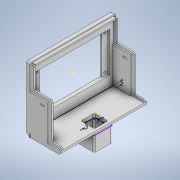
# Autodesk Inventor part: sUPORTE
Saved by Autodesk Inventor 2022 (Build 260153000, 153)
## iProperties
Created: 2022-12-13
Part Number: sUPORTE
Material: Genérico
Document SubType Name: Modeling
Designer: gugarauj07
Density: 1 g/cm^3
Appearance: Padrão
Author: gugarauj07
Autodesk Inventor part; units mm, degrees
ref_plane "YZ Plane" through (0, 0, 0) normal (1, 0, 0) x (0, 1, 0)
ref_plane "XZ Plane" through (0, 0, 0) normal (0, 1, 0) x (-1, 0, 0)
ref_plane "XY Plane" through (0, 0, 0) normal (0, 0, 1) x (1, 0, 0)
sketch "Esboço1" plane through (0, 0, 0) normal (1, 0, 0) x (0, 1, 0)
  line L0 (40.5, 60) -> (-42.5, 60)
  line L1 (-42.5, 60) -> (-42.5, -60)
  line L2 (-42.5, -60) -> (40.5, -60)
  line L3 (42.5, -58) -> (42.5, 58)
  line L4 (-42.5, 60) -> (42.5, -60) construction
  arc A0 (42.5, 58) -> (40.5, 60) centre (40.5, 58) ccw
  arc A1 (40.5, -60) -> (42.5, -58) centre (40.5, -58) ccw
  point P0 (0, 0)
  dimension "d0" = 85
  dimension "d1" = 120
  dimension "d4" = 2
  constraints: 10 end point, 4 point on circle, 4 tangent, 2 centre point, 2 parallel, 2 point on line, 1 equal radius, 1 horizontal, 1 midpoint, 1 perpendicular
  measures "d0" distance of L4.end L1.end
  measures "d1" distance of L0.end L1.end
  measures "d4" radius of A0
extrude "Extrusão1" add sketch "Esboço1" along normal blind 5
sketch "Esboço4" plane through (5, 0, 0) normal (1, 0, 0) x (0, 0, -1)
  line L0 (-60, -42.5) -> (60, -42.5) projected
  line L1 (-60, -42.5) -> (60, -42.5)
  line L2 (60, -42.5) -> (60, -47.5)
  line L3 (60, -47.5) -> (-60, -47.5)
  line L4 (-60, -47.5) -> (-60, -42.5)
  point P0 (0, 0)
  point P1 (60, -42.5)
  dimension "d33" = 5
  constraints: 8 end point, 2 parallel, 1 horizontal, 1 perpendicular
  measures "d33" distance of L1.end L2.end
extrude "Extrusão3" add sketch "Esboço4" against normal blind 5
sketch "Esboço5" plane through (5, 0, 0) normal (1, 0, 0) x (0, 0, -1)
  line L0 (-60, 40.5) -> (-60, -47.5) projected
  line L1 (60, 40.5) -> (60, -47.5) projected
  line L2 (-60, -47.5) -> (60, -47.5)
  line L3 (60, -47.5) -> (60, -42.5)
  line L4 (60, -42.5) -> (-60, -42.5)
  line L5 (-60, -42.5) -> (-60, -47.5)
  point P0 (0, 0)
  point P1 (60, -47.5)
  dimension "d36" = 5
  constraints: 8 end point, 2 parallel, 1 horizontal, 1 perpendicular, 1 point on line
  measures "d36" distance of L3.end L2.end
extrude "Extrusão4" add sketch "Esboço5" along normal blind 43
chamfer "Chanfro2" distance 4 angle 45 1 edges at (0, -47.5, 0)
chamfer "Chanfro3" distance 2 angle 45 1 edges at (48, -47.5, 0)
sketch "Esboço9" plane through (4, -47.5, -60) normal (0, -1, 0) x (1, 0, 0)
  line L0 (23.5, 50.5) -> (38.5, 50.5) projected
  line L1 (31, 50.5) -> (31, 47.5)
  line L2 (38.5, 69.5) -> (23.5, 69.5) projected
  line L3 (31, 69.5) -> (31, 72.5)
  line L4 (43.5, 72.5) -> (16.5, 72.5)
  line L5 (43.5, 47.5) -> (16.5, 47.5)
  line L6 (16.5, 47.5) -> (16.5, 72.5)
  line L7 (43.5, 72.5) -> (43.5, 47.5)
  line L8 (31, 69.5) -> (29.1751, 69.5)
  arc A0 (23.5, 69.5) -> (21.5, 67.5) centre (23.5, 67.5) ccw projected
  line L9 (31, 69.5) -> (23.5, 69.5)
  line L10 (21.5, 67.5) -> (21.5, 52.5) projected
  line L11 (21.5, 67.5) -> (21.5, 52.5)
  arc A1 (21.5, 52.5) -> (23.5, 50.5) centre (23.5, 52.5) ccw projected
  line L12 (23.5, 50.5) -> (31, 50.5)
  line L13 (31, 50.5) -> (38.5, 50.5)
  arc A2 (38.5, 50.5) -> (40.5, 52.5) centre (38.5, 52.5) ccw projected
  line L14 (40.5, 52.5) -> (40.5, 67.5)
  line L15 (38.5, 69.5) -> (31, 69.5)
  arc A3 (38.5, 50.5) -> (40.5, 52.5) centre (38.5, 52.5) ccw
  arc A4 (21.5, 52.5) -> (23.5, 50.5) centre (23.5, 52.5) ccw
  arc A5 (23.5, 69.5) -> (21.5, 67.5) centre (23.5, 67.5) ccw
  arc A6 (40.5, 67.5) -> (38.5, 69.5) centre (38.5, 67.5) ccw projected
  arc A7 (40.5, 67.5) -> (38.5, 69.5) centre (38.5, 67.5) ccw
  point P0 (-4, 60)
  dimension "d103" = 3
  dimension "d104" = 3
  constraints: 26 end point, 8 point on circle, 5 vertical, 4 centre point, 4 tangent, 3 collinear, 2 midpoint, 2 perpendicular, 1 horizontal, 1 point on line
  measures "d103" distance of L1.start L1.end
  measures "d104" distance of L3.start L3.end
extrude "Extrusão7" add sketch "Esboço9" along normal blind 21 contours L0 L1 L5 L6 L4 L3 L2 A0 L10 A1
extrude "Extrusão9" add sketch "Esboço9" along normal blind 21 contours L0 A2 L14 A6 L2 L3 L4 L7 L5 L1
fillet "Arredondamento1" radius 2 4 edges at (47.5, -58, -12.5) (20.5, -58, -12.5) (20.5, -58, 12.5) (47.5, -58, 12.5)
sketch "Esboço12" plane through (5, 0, 0) normal (1, 0, 0) x (0, 0, -1)
  line L0 (60, -42.5) -> (60, 40.5) projected
  line L1 (60, -42.5) -> (55, -42.5)
  line L2 (55, -42.5) -> (55, 7.5)
  line L3 (55, 7.5) -> (60, 7.5)
  line L4 (60, 7.5) -> (60, -42.5)
  line L5 (60, -42.5) -> (-60, -42.5) projected
  line L6 (-60, -42.5) -> (-55, -42.5)
  line L7 (-55, -42.5) -> (-55, 7.5)
  line L8 (-55, 7.5) -> (-60, 7.5)
  line L9 (-60, 7.5) -> (-60, -42.5)
  point P0 (0, 0)
  dimension "d123" = 5
  dimension "d124" = 50
  dimension "d125" = 5
  dimension "d126" = 50
  constraints: 16 end point, 4 parallel, 2 horizontal, 2 perpendicular
  measures "d123" distance of L2.end L3.end
  measures "d124" distance of L1.end L2.end
  measures "d125" distance of L8.end L7.end
  measures "d126" distance of L7.end L6.end
extrude "Extrusão10" add sketch "Esboço12" along normal blind 25
sketch "Esboço13" plane through (30, 0, 0) normal (1, 0, 0) x (0, 0, -1)
  line L0 (-60, 40.5) -> (-60, -43.5) projected
  line L1 (-60, -42.5141) -> (-58.5, -42.5141)
  line L2 (-60, -42.5141) -> (-58.5, -42.5141) construction
  line L3 (60, -42.5) -> (-60, -42.5) projected
  line L4 (-55, 7.5) -> (-60, 7.5) projected
  line L5 (-58.5, -42.5) -> (-56.5, -42.5)
  line L6 (-56.5, -42.5) -> (-56.5, 7.5)
  line L7 (-56.5, 7.5) -> (-58.5, 7.5)
  line L8 (-58.5, 7.5) -> (-58.5, -42.5)
  line L9 (58, 42.5) -> (-58, 42.5) projected
  line L10 (-57.5, 42.5) -> (-56, 42.5) construction
  line L11 (-58.5, 7.5) -> (-56.5, 7.5)
  line L12 (60, -42.5) -> (55, -42.5) projected
  line L13 (60, -42.5) -> (58.5, -42.5)
  line L14 (55, 7.5) -> (60, 7.5) projected
  line L15 (58.5, -42.5) -> (56.5, -42.5)
  line L16 (56.5, -42.5) -> (56.5, 7.5)
  line L17 (56.5, 7.5) -> (58.5, 7.5)
  line L18 (58.5, 7.5) -> (58.5, -42.5)
  point P0 (0, 0)
  dimension "d129" = 1.5
  dimension "d130" = 0
  dimension "d135" = 1.5
  dimension "d136" = 2
  constraints: 26 end point, 6 point on line, 5 horizontal, 4 parallel, 3 perpendicular, 1 collinear
  measures "d129" distance of L1.start L1.end
  measures "d130" distance between parallel lines of L1 L2
  measures "d135" distance of L3.start L13.end
  measures "d136" distance of L16.end L17.end
extrude "Extrusão11" add sketch "Esboço13" along normal blind 4 contours L4 L6 L3 L8 | L3 L16 L14 L18
extrude "Extrusão12" cut sketch "Esboço9" against normal blind 6 contours A1 L10 A0 L2 A6 L14 A2 L0
sketch "Esboço14" plane through (5, 0, 0) normal (1, 0, 0) x (0, 0, -1)
  line L0 (-58.5, 7.5) -> (-60, 7.5) projected
  line L1 (-58.5, 7.5) -> (-56.5, 7.5)
  line L2 (-56.5, 7.5) -> (-56.5, 41)
  line L3 (-56.5, 41) -> (-56.5, 41)
  line L4 (-58.5, 39) -> (-58.5, 7.5)
  line L5 (55, 7.5) -> (60, 7.5) projected
  line L6 (58.5055, 7.5) -> (56.5055, 7.5)
  line L7 (56.5055, 7.5) -> (56.5055, 41)
  line L8 (56.5055, 41) -> (56.5055, 41)
  line L9 (58.5055, 39) -> (58.5055, 7.5)
  line L10 (-56.5, 41) -> (56.5055, 41)
  line L11 (56.5055, 41) -> (56.5055, 39)
  line L12 (56.5055, 39) -> (-56.5, 39)
  line L13 (-56.5, 39) -> (-56.5, 41)
  arc A0 (-56.5, 41) -> (-58.5, 39) centre (-56.5, 39) ccw
  arc A1 (58.5055, 39) -> (56.5055, 41) centre (56.5055, 39) ccw
  point P0 (0, 0)
  point P1 (-58.5, 41)
  point P2 (58.5055, 41)
  dimension "d141" = 2
  dimension "d142" = 33.5
  dimension "d143" = 2
  dimension "d144" = 33.5
  dimension "d145" = 2
  dimension "d146" = 2
  dimension "d147" = 2
  constraints: 24 end point, 6 parallel, 6 point on line, 4 point on circle, 4 tangent, 3 horizontal, 3 perpendicular, 2 centre point
  measures "d141" distance of point (-58.5, 41) L2.end
  measures "d142" distance of L2.end L1.end
  measures "d143" distance of L7.end point (58.505, 41)
  measures "d144" distance of L6.end L7.end
  measures "d145" distance of L10.end L11.end
  measures "d146" radius of A0
  measures "d147" radius of A1
extrude "Extrusão13" add sketch "Esboço14" along normal blind 4
sketch "Esboço15" plane through (9, 0, 0) normal (1, 0, 0) x (0, 0, -1)
  line L0 (-56.5, 7.5) -> (-56.5, 39) projected
  line L1 (-56.5, 7.5) -> (-58.5, 7.5)
  line L2 (-58.5, 7.5) -> (-58.5, 10.5)
  line L3 (-58.5, 10.5) -> (-56.5, 10.5)
  line L4 (-56.5, 10.5) -> (-56.5, 7.5)
  line L5 (58.5, 7.5) -> (56.5, 7.5) projected
  line L6 (56.5055, 39) -> (56.5055, 7.5) projected
  line L7 (58.5, 7.5) -> (56.5055, 7.5)
  line L8 (56.5055, 7.5) -> (56.5055, 10.5)
  line L9 (56.5055, 10.5) -> (58.5, 10.5)
  line L10 (58.5, 10.5) -> (58.5, 7.5)
  point P0 (0, 0)
  dimension "d150" = 2
  dimension "d151" = 3
  dimension "d152" = 3
  constraints: 16 end point, 4 parallel, 2 horizontal, 2 perpendicular, 1 point on line
  measures "d150" distance of L2.end L3.end
  measures "d151" distance of L1.end L2.end
  measures "d152" distance of L7.end L8.end
extrude "Extrusão14" add sketch "Esboço15" along normal blind 25
sketch "Esboço16" plane through (34, 0, 0) normal (1, 0, 0) x (0, 0, -1)
  line L0 (-56.5, -42.5) -> (-58.5, -42.5) projected
  line L1 (-58.5, -42.5) -> (-58.5, 7.5) projected
  line L2 (-56.5, -42.5) -> (-58.5, -42.5)
  line L3 (-58.5, -42.5) -> (-58.5, -39.5)
  line L4 (-58.5, -39.5) -> (-56.5, -39.5)
  line L5 (-56.5, -39.5) -> (-56.5, -42.5)
  line L6 (60, -42.5) -> (58.5, -42.5) projected
  line L7 (58.5, -42.5) -> (56.5, -42.5)
  line L8 (56.5, -42.5) -> (56.5, -39.5)
  line L9 (56.5, -39.5) -> (58.5, -39.5)
  line L10 (58.5, -39.5) -> (58.5, -42.5)
  point P0 (0, 0)
  dimension "d155" = 3
  dimension "d156" = 2
  dimension "d157" = 3
  constraints: 16 end point, 4 parallel, 2 horizontal, 2 perpendicular, 1 point on line
  measures "d155" distance of L2.end L3.end
  measures "d156" distance of L8.end L9.end
  measures "d157" distance of L7.end L8.end
extrude "Extrusão15" add sketch "Esboço16" along normal blind 14
chamfer "Chanfro4" distance 2 angle 45 2 edges at (48, -39.5, 57.5) (48, -39.5, -57.5)
chamfer "Chanfro5" distance 2 angle 45 2 edges at (34, 10.5, 57.5) (34, 10.5, -57.5027)
sketch "Esboço17" plane through (9, 0, 0) normal (1, 0, 0) x (0, 0, -1)
  line L0 (-60, 42.5) -> (-57, 42.5)
  line L1 (-57, 42.5) -> (-57, 39.5)
  line L2 (-57, 39.5) -> (-60, 39.5)
  line L3 (-60, 39.5) -> (-60, 42.5)
  line L4 (60, 42.5) -> (57, 42.5)
  line L5 (57, 42.5) -> (57, 39.5)
  line L6 (57, 39.5) -> (60, 39.5)
  line L7 (60, 39.5) -> (60, 42.5)
  point P0 (0, 0)
  dimension "d166" = 3
  dimension "d167" = 3
  dimension "d168" = 3
  dimension "d169" = 3
  constraints: 16 end point, 4 parallel, 2 horizontal, 2 perpendicular
  measures "d166" distance of L1.end L2.end
  measures "d167" distance of L0.end L1.end
  measures "d168" distance of L6.end L5.end
  measures "d169" distance of L5.end L4.end
hole "Furo5" at (9, 39.5, 57) at (9, 39.5, -57) direction (-1, 0, 0) diameter 3.302 depth 12.3 tip angle 118 thread size "8-32 UNC" class "2B" standard "ANSI Unified Screw Threads"
sketch "Esboço18" plane through (4, -68.5, -60) normal (0, -1, 0) x (1, 0, 0)
  line L0 (21.5, 102.5) -> (21.5, 87.5) projected
  line L1 (21.5, 102.5) -> (21.5, 101.5)
  line L2 (21.5, 101.5) -> (19.5, 101.5)
  line L3 (19.5, 101.5) -> (19.5, 88.5)
  line L4 (19.5, 88.5) -> (21.5, 88.5)
  line L5 (21.5, 88.5) -> (21.5, 101.5)
  arc A0 (23.5, 69.5) -> (21.5, 67.5) centre (23.5, 67.5) ccw projected
  line L6 (21.5, 67.5) -> (21.5, 66.5)
  line L7 (21.5, 67.5) -> (21.5, 52.5) projected
  line L8 (21.5, 66.5) -> (19.5, 66.5)
  line L9 (19.5, 66.5) -> (19.5, 53.5)
  line L10 (19.5, 53.5) -> (21.5, 53.5)
  line L11 (21.5, 53.5) -> (21.5, 66.5)
  line L12 (21.5, 32.5) -> (21.5, 17.5) projected
  line L13 (21.5, 32.5) -> (21.5, 31.5)
  line L14 (21.5, 31.5) -> (19.5, 31.5)
  line L15 (19.5, 31.5) -> (19.5, 18.5)
  line L16 (19.5, 18.5) -> (21.5, 18.5)
  line L17 (21.5, 18.5) -> (21.5, 31.5)
  point P0 (-4, 60)
  point P1 (21.5, 18.5)
  dimension "d177" = 1
  dimension "d178" = 2
  dimension "d179" = 13
  dimension "d180" = 1
  dimension "d181" = 2
  dimension "d182" = 13
  dimension "d183" = 1
  dimension "d184" = 13
  constraints: 30 end point, 6 parallel, 3 horizontal, 3 perpendicular, 3 point on line
  measures "d177" distance of L0.start L1.end
  measures "d178" distance of L4.end L3.end
  measures "d179" distance of L3.end L2.end
  measures "d180" distance of L6.start L6.end
  measures "d181" distance of L10.end L9.end
  measures "d182" distance of L9.end L8.end
  measures "d183" distance of L12.start L13.end
  measures "d184" distance of L15.end L14.end
extrude "Extrusão16" cut sketch "Esboço18" against normal blind 19
sketch "Esboço21" plane through (0, 40.5, 60) normal (0, 0, 1) x (1, 0, 0)
  line L0 (20, -41) -> (25, -41)
  line L1 (25, -41) -> (25, -39)
  line L2 (25, -39) -> (20, -39)
  line L3 (20, -39) -> (20, -41)
  point P0 (0, -40.5)
  point P1 (30, -33)
  dimension "d195" = 5
  dimension "d196" = 2
  constraints: 8 end point, 2 parallel, 1 horizontal, 1 perpendicular
  measures "d195" distance of L2.end L1.end
  measures "d196" distance of L1.end L0.end
extrude "Extrusão18" cut sketch "Esboço21" against normal through all
sketch "Esboço22" plane through (5, 0, 0) normal (1, 0, 0) x (0, 0, -1)
  line L0 (43.5, -28) -> (-43.5, -28)
  line L1 (-43.5, -28) -> (-43.5, 28)
  line L2 (-43.5, 28) -> (43.5, 28)
  line L3 (43.5, 28) -> (43.5, -28)
  line L4 (43.5, -28) -> (-43.5, 28) construction
  line L5 (-43.5, -28) -> (43.5, 28) construction
  point P0 (0, 0)
  dimension "d199" = 87
  dimension "d200" = 56
  constraints: 12 end point, 2 midpoint, 2 parallel, 1 horizontal, 1 perpendicular
  measures "d199" distance of L1.end L2.end
  measures "d200" distance of L0.end L1.end
extrude "Extrusão19" cut sketch "Esboço22" against normal through all
sketch "Esboço23" plane through (5, 0, 0) normal (1, 0, 0) x (0, 0, -1)
  line L0 (-43.5, -28) -> (-43.5, 28) projected
  line L1 (-43.5, 28) -> (-51.5, 28)
  line L2 (-51.5, 28) -> (-51.5, -28)
  line L3 (-51.5, -28) -> (-43.5, -28)
  line L4 (-43.5, -28) -> (-43.5, 28)
  line L5 (43.5, 28) -> (43.5, -28) projected
  line L6 (43.5, -28) -> (51.5, -28)
  line L7 (51.5, -28) -> (51.5, 28)
  line L8 (51.5, 28) -> (43.5, 28)
  line L9 (43.5, 28) -> (43.5, -28)
  point P0 (0, 0)
  dimension "d203" = 8
  dimension "d204" = 8
  constraints: 16 end point, 4 parallel, 2 horizontal, 2 perpendicular, 1 point on line
  measures "d203" distance of L3.end L2.end
  measures "d204" distance of L8.end L7.end
extrude "Extrusão20" cut sketch "Esboço23" against normal blind 3
sketch "Esboço24" plane through (2, 0, 0) normal (1, 0, 0) x (0, 0, -1)
  line L0 (51.5, -28) -> (-51.5, -28) projected
  line L1 (-51.5, -28) -> (-47.5, -28)
  circle A0 centre (-47.5, -24) radius 1.5
  line L2 (-43.5, -28) -> (43.5, -28) projected
  line L3 (43.5, 28) -> (-43.5, 28) projected
  circle A1 centre (47.5, -24) radius 1.5
  line L4 (-51.5, -28) -> (-51.5, 28) projected
  line L5 (51.5, 28) -> (51.5, -28) projected
  circle A2 centre (-47.5, 24) radius 1.5
  circle A3 centre (47.5, 24) radius 1.5
  dimension "d209" = 3
  constraints: 4 centre point, 2 end point, 1 horizontal
  measures "d209" diameter of A0
extrude "Extrusão21" cut sketch "Esboço24" against normal through all
